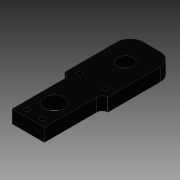
# Autodesk Inventor part: Fixture_Airpot_Support
Saved by Autodesk Inventor 2015 (Build 190159000, 159)
## iProperties
Created: 2014-12-16
Part Number: Fixture_Airpot_Support
Material: Generic
Document SubType Name: Modeling
Designer: amarschn
Density: 1 g/cm^3
Appearance: Anodized - Black
Author: amarschn
Autodesk Inventor part; units mm, degrees
ref_plane "YZ Plane" through (0, 0, 0) normal (1, 0, 0) x (0, 1, 0)
ref_plane "XZ Plane" through (0, 0, 0) normal (0, 1, 0) x (-1, 0, 0)
ref_plane "XY Plane" through (0, 0, 0) normal (0, 0, 1) x (1, 0, 0)
sketch "Sketch1" plane through (0, 0, 0) normal (0, 1, 0) x (-1, 0, 0)
  line L0 (15.5575, -22.86) -> (15.5575, 27.94)
  line L1 (15.5575, 27.94) -> (-15.5575, 27.94)
  line L2 (-15.5575, 27.94) -> (-15.5575, -22.86)
  line L3 (-15.5575, -27.94) -> (15.5575, 27.94) construction
  line L4 (15.5575, -27.94) -> (-15.5575, 27.94) construction
  line L5 (20.6375, -27.94) -> (20.955, -27.94)
  line L6 (20.955, -27.94) -> (20.955, -78.74)
  line L7 (8.255, -91.44) -> (-8.255, -91.44)
  line L8 (-20.955, -78.74) -> (-20.955, -27.94)
  line L9 (-20.955, -27.94) -> (-20.6375, -27.94)
  arc A0 (15.5575, -22.86) -> (20.6375, -27.94) centre (20.6375, -22.86) ccw
  arc A1 (-20.6375, -27.94) -> (-15.5575, -22.86) centre (-20.6375, -22.86) ccw
  circle A2 centre (0, 2.54) radius 9.525
  arc A3 (8.255, -91.44) -> (20.955, -78.74) centre (8.255, -78.74) ccw
  arc A4 (-20.955, -78.74) -> (-8.255, -91.44) centre (-8.255, -78.74) ccw
  circle A5 centre (0, -66.04) radius 7.366
  line L10 (0, 46.0525) -> (0, -103.086)
  circle A6 centre (7.62, 21.59) radius 2.3813
  circle A7 centre (-7.62, 21.59) radius 2.3813
  circle A8 centre (12.5412, -34.29) radius 2.3813
  circle A9 centre (-12.5412, -34.29) radius 2.3813
  point P0 (0, 0)
  point P1 (20.955, -91.44)
  point P2 (-20.955, -91.44)
  point P3 (0, 0)
  dimension "d0" = 5.08
  dimension "d1" = 31.115
  dimension "d2" = 41.91
  dimension "d3" = 63.5
  dimension "d4" = 119.38
  dimension "d5" = 19.05
  dimension "d6" = 25.4
  dimension "d7" = 12.7
  dimension "d27" = 25.4
  dimension "d28" = 14.732
  dimension "d29" = 4.7625
  dimension "d30" = 15.24
  dimension "d31" = 6.35
  dimension "d32" = 25.0825
  dimension "d33" = 4.7625
  dimension "d34" = 57.15
  constraints: 22 end point, 12 point on line, 10 centre point, 8 point on circle, 8 tangent, 4 perpendicular, 3 midpoint, 2 equal radius, 2 symmetric about line, 1 collinear, 1 horizontal, 1 parallel, 1 vertical, 3 other
  measures "d0" radius of A0
  measures "d1" distance of L0.end L1.end
  measures "d2" distance of point (20.955, -91.44) point (-20.955, -91.44)
  measures "d3" distance of L5.end point (20.955, -91.44)
  measures "d4" distance between parallel lines of L7 L1
  measures "d5" diameter of A2
  measures "d6" distance from line of L1 A2.centre
  measures "d7" radius of A3
  measures "d27" distance from line of L7 A5.centre
  measures "d28" diameter of A5
  measures "d29" diameter of A6
  measures "d30" distance of A7.centre A6.centre
  measures "d31" distance from line of L1 A6.centre
  measures "d32" distance of A9.centre A8.centre
  measures "d33" diameter of A8
  measures "d34" distance from line of L7 A8.centre
extrude "Extrusion1" add sketch "Sketch1" along normal blind 12.7 contours A0 L5 L6 A3 L7 L10 A5 A2 L1 L0 | L10 A2 A5 L7 A4 L8 L9 A1 L2 L1
sketch "Sketch4" plane through (0, 0, 0) normal (0, -1, 0) x (1, 0, 0)
  circle A0 centre (0, -66.04) radius 7.366 projected
  circle A1 centre (0, -66.04) radius 19.05
  point P0 (0, 0)
  dimension "d38" = 38.1
  constraints: 1 centre point, 1 coincident
  measures "d38" diameter of A1
extrude "Extrusion3" cut sketch "Sketch4" against normal blind 2.54
equation "\"d33\" = d29"
body "Solid1"
